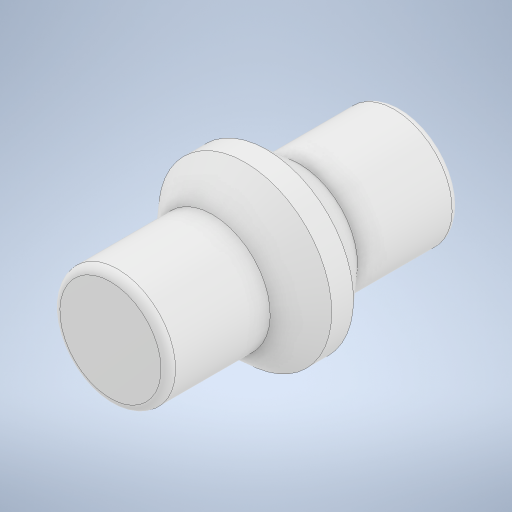
# Autodesk Inventor part: RailPlug
Saved by Autodesk Inventor 2023.1 (Build 271208000, 208)
## iProperties
Created: 2023-06-05
Part Number: RailPlug
Material: ABS Plastic
Document SubType Name: Modeling
Designer: hello
Density: 1.06 g/cm^3
Appearance: Smooth - White
Author: hello
Autodesk Inventor part; units mm, degrees
ref_plane "YZ Plane" through (0, 0, 0) normal (1, 0, 0) x (0, 1, 0)
ref_plane "XZ Plane" through (0, 0, 0) normal (0, 1, 0) x (-1, 0, 0)
ref_plane "XY Plane" through (0, 0, 0) normal (0, 0, 1) x (1, 0, 0)
sketch "Sketch1" plane through (0, 0, 0) normal (1, 0, 0) x (0, 1, 0)
  line L0 (0, 0) -> (0, -20)
  line L1 (0, 0) -> (3.975, 0)
  line L2 (3.975, 0) -> (3.975, -7)
  line L3 (3.975, -7) -> (5.95, -9.25)
  line L4 (5.95, -9.25) -> (5.95, -10.75)
  line L5 (5.95, -10.75) -> (3.975, -13)
  line L6 (3.975, -13) -> (3.975, -20)
  line L7 (3.975, -20) -> (0, -20)
  dimension "d0" = 7.95
  dimension "d1" = 20
  dimension "d2" = 6
  dimension "d3" = 1.5
  dimension "d4" = 11.9
  constraints: 16 end point, 2 equal length, 2 perpendicular, 2 vertical, 1 horizontal, 1 parallel, 1 vertical alignment
  measures "d0" diameter of L2 L0
  measures "d1" distance of L0.start L0.end
  measures "d2" distance of L5.end L2.end
  measures "d3" distance of L3.end L4.end
  measures "d4" diameter of L4 L0
revolve "Revolution1" add sketch "Sketch1" angle 360 about axis through (0, 0, 0) along (0, 0, -1)
fillet "Fillet1" radius 0.5 2 edges at (0, -3.975, 0) (0, -3.975, -20)
body "Solid1"
